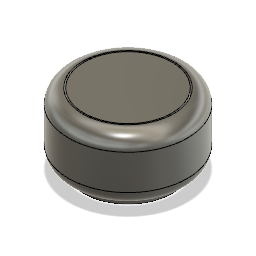
dupla_mainbody v2 (Autodesk Fusion 360 design; units mm, degrees)
Autodesk Fusion 360 part; units mm, degrees
sketch "Sketch2" plane through (0, 0, 0) normal (0, 1, 0) x (1, 0, 0) in component "Component"
  circle A0 centre (0, 0) radius 32.5
  circle A1 centre (0, 0) radius 42.5
  circle A2 centre (0, 0) radius 31.5
  dimension "d17" = 65
  dimension "d18" = 85
  dimension "d19" = 63
  constraint coincident A0.centre A1.centre
  constraint concentric A1 A2
  measures "d17" diameter of A0
  measures "d18" diameter of A1
  measures "d19" diameter of A2
extrude "Extrude5" add sketch "Sketch2" along normal blind 15 contours A2 makes body 1 in component "Component"
extrude "Extrude6" add sketch "Sketch2" along normal blind 10 separate body contours A1 makes body 2 in component "Component"
move_body "Move2" bodies 2 to x (1, 0, 0) y (0, 1, 0) z (0, 0, 1) at (0, 5, 0) in component "Component"
copy_body "CopyPasteBodies2" bodies 2 makes body 3 in component "Component"
move_body "Move3" bodies 3 to x (1, 0, 0) y (0, 1, 0) z (0, 0, 1) at (0, 35, 0) in component "Component"
copy_body "CopyPasteBodies3" bodies 1 makes body 4 in component "Component"
move_body "Move4" bodies 4 to x (1, 0, 0) y (0, 1, 0) z (0, 0, 1) at (0, 35, 0) in component "Component"
fillet "Fillet2" radius 10 2 edges at (-39.6239, 5, 15.3687) (-39.6239, 50, 15.3687) on bodies 2 3 in component "Component"
extrude "Extrude7" add sketch "Sketch2" along normal blind 40 separate body contours A1 makes body 5 in component "Component"
extrude "Extrude8" cut sketch "Sketch2" 1 faces at (38.8874, 0, 3.7261) against normal blind 15 contours A1 on bodies 5 bodies 2 5 in component "Component"
extrude "Extrude9" cut 1 faces at (38.8874, 0, 3.7261) along direction (0, 1, 0) blind 15 on bodies 5 bodies 5 in component "Component"
component "Component" placed x (1, 0, 0) y (0, 1, 0) z (0, 0, 1) at (0, 0, 0)
named bodies: "Base", "BottomFilet", "TopFilet", "TopLEDScreen", "SideSpeaker+Mic"
